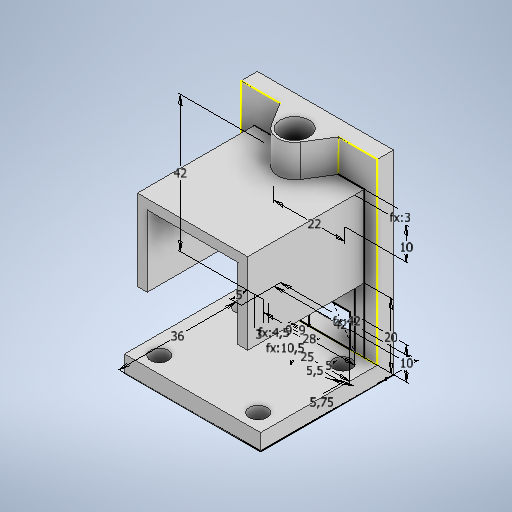
# Autodesk Inventor part: KatownikNowy
Saved by Autodesk Inventor 2025 (Build 290162000, 162)
## iProperties
Created: 2024-09-20
Part Number: KatownikNowy
Material: Ogólny
Document SubType Name: Modeling
Designer: user
Density: 1 g/cm^3
Appearance: Domyślna
Author: user
Autodesk Inventor part; units mm, degrees
ref_plane "YZ Plane" through (0, 0, 0) normal (1, 0, 0) x (0, 1, 0)
ref_plane "XZ Plane" through (0, 0, 0) normal (0, 1, 0) x (-1, 0, 0)
ref_plane "XY Plane" through (0, 0, 0) normal (0, 0, 1) x (1, 0, 0)
sketch "Szkic1" plane through (0, 0, 0) normal (0, 1, 0) x (-1, 0, 0)
  line L0 (-21, 18) -> (21, 18)
  line L1 (21, 18) -> (21, -18)
  line L2 (21, -18) -> (-21, -18)
  line L3 (-21, -18) -> (-21, 18)
  line L4 (-21, 18) -> (21, -18) construction
  line L5 (21, 18) -> (-21, -18) construction
  circle A0 centre (-15.25, -13) radius 2.75
  line L6 (0, 18) -> (0, -18)
  line L7 (-21, 0) -> (21, 0)
  circle A1 centre (-15.25, 13) radius 2.75
  line L8 (0, -18) -> (0, 18)
  circle A2 centre (15.25, -13) radius 2.75
  circle A3 centre (15.25, 13) radius 2.75
  line L9 (-21, -18) -> (20.4575, -18)
  line L10 (-21, -18) -> (21, -18)
  line L11 (21, -18) -> (21, -23)
  line L12 (21, -23) -> (-21, -23)
  line L13 (-21, -23) -> (-21, -18)
  circle A4 centre (0, -13.5) radius 4.5
  circle A5 centre (0, -13.5) radius 5.25
  line L14 (9, -18) -> (4.453, -10.7191)
  line L15 (-9, -18) -> (-4.453, -10.7191)
  point P0 (0, 0)
  point P1 (-21, -20.5)
  point P2 (0, -18)
  dimension "d11" = 10.5
  dimension "W12" = 42
  dimension "L12" = 36
  dimension "d2" = 5.5
  dimension "d3" = 5.75
  dimension "d4" = 5
  dimension "d6" = 5
  dimension "d7" = 42
  dimension "SrPopr" = 9
  dimension "d9" = 4.5
  dimension "d12" = 9
  constraints: 32 end point, 8 midpoint, 7 symmetric about line, 5 centre point, 4 parallel, 3 horizontal, 2 perpendicular, 2 point on line, 1 coincident, 7 other
  measures "W12" distance of L1.end L2.end
  measures "L12" distance of L0.end L1.end
  measures "d2" diameter of A0
  measures "d3" distance from line of L3 A0.centre
  measures "d4" distance from line of L2 A0.centre
  measures "d6" distance of L10.end L11.end
  measures "d7" distance from line of point (-21, -20.5) L11
  measures "SrPopr" diameter of A4
  measures "d9" distance from line of L9 A4.centre
  measures "d12" distance from line of L8 L14.start
extrude "Wyciągnięcie proste1" add sketch "Szkic1" along normal blind 5
extrude "Wyciągnięcie proste2" add sketch "Szkic1" along normal blind 60 contours L2 A5 L11 L12 L13 | A5 L2 A4 L6 | L6 A4 L2 A5 | L15 A5 L2 | L14 L2 A5 | L2 A5
extrude "Wyciągnięcie proste3" cut sketch "Szkic1" along normal blind 50 contours A5 L2 A4 L6 | L6 A4 L2 A5 | L15 A5 L2 | L14 L2 A5
extrude "Wyciągnięcie proste4" add sketch "Szkic1" along normal blind 5 contours A5 L2 A4 L6 | L6 A4 L2 A5 | L15 A5 L2 | L14 L2 A5
sketch "Szkic3" plane through (-21, 5, -18) normal (0, 0, 1) x (1, 0, 0)
  line L0 (42, 0) -> (0, 0) projected
  line L1 (42, 0) -> (42, 55) projected
  line L2 (30, 55) -> (42, 55) projected
  line L3 (30, 45) -> (30, 55) projected
  line L4 (30, 45) -> (21, 45) projected
  line L5 (21, 45) -> (12, 45) projected
  line L6 (12, 45) -> (12, 55) projected
  line L7 (0, 55) -> (12, 55) projected
  line L8 (0, 0) -> (0, 55) projected
  line L9 (35, 42) -> (7, 42)
  line L10 (7, 42) -> (7, 0)
  line L11 (7, 0) -> (35, 0)
  line L12 (35, 0) -> (35, 42)
  line L13 (35, 42) -> (7, 0) construction
  line L14 (7, 42) -> (35, 0) construction
  line L15 (42, 0) -> (42, 55) projected
  line L16 (0, 0) -> (0, 55) projected
  line L17 (0, 0) -> (42, 0) projected
  line L18 (21, 0) -> (21, 42)
  line L19 (38, 0) -> (38, 45)
  line L20 (4, 45) -> (4, 0)
  line L21 (38, 45) -> (4, 45)
  line L22 (33.5, 0) -> (8.5, 0)
  line L23 (8.5, 0) -> (8.5, 10)
  line L24 (8.5, 10) -> (33.5, 10)
  line L25 (33.5, 10) -> (33.5, 0)
  line L26 (32, 42) -> (10, 42)
  line L27 (10, 42) -> (10, 32)
  line L28 (10, 32) -> (32, 32)
  line L29 (32, 32) -> (32, 42)
  line L30 (38, 20) -> (4, 20)
  point P0 (21, -5)
  point P1 (21, 21)
  point P2 (21, 0)
  point P3 (4, 0)
  point P4 (38, 0)
  point P5 (8.5, 0)
  point P6 (33.5, 0)
  point P7 (35, 20)
  point P8 (7, 20)
  dimension "d21" = 28
  dimension "d22" = 42
  dimension "GruboscAku" = 3
  dimension "d33" = 3
  dimension "d34" = 10
  dimension "d35" = 25
  dimension "d36" = 10
  dimension "d37" = 22
  dimension "d42" = 20
  constraints: 38 end point, 9 parallel, 8 point on line, 5 midpoint, 4 perpendicular, 2 horizontal, 1 coincident, 1 collinear, 4 other
  measures "d21" distance of L11.end L10.end
  measures "d22" distance of L10.end L9.end
  measures "GruboscAku" distance between parallel lines of L10 L20
  measures "d33" distance between parallel lines of L9 L21
  measures "d34" distance between parallel lines of L22 L24
  measures "d35" distance between parallel lines of L23 L25
  measures "d36" distance between parallel lines of L28 L9
  measures "d37" distance between parallel lines of L27 L29
  measures "d42" distance between parallel lines of L0 L30
extrude "Wyciągnięcie proste5" add sketch "Szkic3" along normal blind 36 contours L30 L12 L9 L10 L20 L21 L5 L4 L19
extrude "Wyciągnięcie proste6" cut sketch "Szkic3" against normal blind 5 contours L0 L18 L24 L25 | L0 L23 L24 L18 | L29 L28 L18 L9 | L28 L27 L9 L18
extrude "Wyciągnięcie proste7" cut sketch "Szkic1" along normal blind 50 contours A4 L6 | L6 A4
extrude "Wyciągnięcie proste8" add sketch "Szkic1" along normal blind 5 contours A4 L6 | L6 A4
equation "\"d7\" = W12"
equation "\"d9\" = 0.5 * SrPopr"
equation "\"d33\" = GruboscAku"
